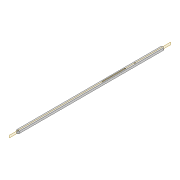
# Autodesk Inventor part: Part_11
Saved by Autodesk Inventor 2022 (Build 260153000, 153)
## iProperties
Created: 2022-05-03
Part Number: Part_11
Material: Generic
Document SubType Name: Modeling
Designer: dell
Density: 1 g/cm^3
Appearance: Default
Author: dell
Autodesk Inventor part; units mm, degrees
ref_plane "XZ Plane" through (0, 0, 0) normal (0, 1, 0) x (-1, 0, 0)
ref_plane "XY Plane" through (0, 0, 0) normal (0, 0, 1) x (1, 0, 0)
sketch "Sketch1" plane through (0, 0, 0) normal (0, 1, 0) x (-1, 0, 0)
  line L0 (0, 0) -> (0, -343.336) construction
  line L1 (-4, 0) -> (-4, -343.336)
  line L2 (4, -343.336) -> (4, 0)
  arc A0 (4, 0) -> (-4, 0) centre (0, 0) ccw
  arc A1 (-4, -343.336) -> (4, -343.336) centre (0, -343.336) ccw
  circle A2 centre (0, 0) radius 1.5
  circle A3 centre (0, -343.336) radius 1.5
  line L3 (0, -315.436) -> (0, -248.336) construction
  line L4 (1.5, -315.436) -> (1.5, -248.336)
  line L5 (-1.5, -248.336) -> (-1.5, -315.436)
  arc A4 (-1.5, -315.436) -> (1.5, -315.436) centre (0, -315.436) ccw
  arc A5 (1.5, -248.336) -> (-1.5, -248.336) centre (0, -248.336) ccw
  line L6 (0, -343.336) -> (0, -423.336) construction
  line L7 (-4, -343.336) -> (-4, -423.336)
  line L8 (4, -423.336) -> (4, -343.336)
  arc A6 (4, -343.336) -> (-4, -343.336) centre (0, -343.336) ccw
  arc A7 (-4, -423.336) -> (4, -423.336) centre (0, -423.336) ccw
  point P0 (0, -171.668)
  point P1 (0, -281.886)
  point P2 (0, -383.336)
  dimension "d0" = 8
  dimension "d1" = 343.336
  dimension "d2" = 3
  dimension "d3" = 3
  dimension "d14" = 3
  dimension "d15" = 27.9
  dimension "d16" = 95
  dimension "d17" = 8
  dimension "d18" = 80
  constraints: 24 end point, 12 point on circle, 12 tangent, 8 centre point, 3 midpoint, 3 parallel, 3 point on line, 2 coincident, 1 vertical
  measures "d0" diameter of A1
  measures "d1" distance of L0.end L0.start
  measures "d2" diameter of A2
  measures "d3" diameter of A3
  measures "d14" diameter of A5
  measures "d15" distance of L0.end L3.start
  measures "d16" distance of L0.end L3.end
  measures "d17" diameter of A7
  measures "d18" distance of L6.end L0.end
extrude "Extrusion1" add sketch "Sketch1" along normal blind 6
sketch "Sketch3" plane through (0, 6, 0) normal (0, 1, 0) x (1, 0, 0)
  line L0 (-4, 423.336) -> (-4, 0) projected
  line L1 (-4, 214.6062) -> (0, 206.0281)
  line L2 (0, 206.0281) -> (4, 214.6062)
  line L3 (4, 0) -> (4, 423.336) projected
  line L4 (-4, 423.336) -> (-4, 0) projected
  arc A0 (-4, 0) -> (4, 0) centre (0, 0) ccw projected
  line L5 (4, 0) -> (4, 423.336) projected
  arc A1 (4, 423.336) -> (-4, 423.336) centre (0, 423.336) ccw projected
  arc A2 (1.5, 315.436) -> (-1.5, 315.436) centre (0, 315.436) ccw projected
  line L6 (1.5, 315.436) -> (1.5, 248.336) projected
  arc A3 (-1.5, 248.336) -> (1.5, 248.336) centre (0, 248.336) ccw projected
  line L7 (-1.5, 248.336) -> (-1.5, 315.436) projected
  circle A4 centre (0, 343.336) radius 1.5 projected
  circle A5 centre (0, 0) radius 1.5 projected
  dimension "d21" = 25
  dimension "d22" = 25
  constraints: 4 end point, 2 point on line
  measures "d21" angle of L3 L2
  measures "d22" angle of L0 L1
extrude "Extrusion2" [suppressed]
body "Solid1"
